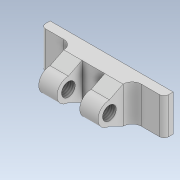
# Autodesk Inventor part: dobradicaP1
Saved by Autodesk Inventor 2020.4 (Build 244396000, 396)
## iProperties
Created: 2021-05-31
Part Number: dobradicaP1
Material: Generic
Document SubType Name: Modeling
Designer: becca
Density: 1 g/cm^3
Appearance: Default
Author: becca
Autodesk Inventor part; units mm, degrees
ref_plane "YZ Plane" through (0, 0, 0) normal (1, 0, 0) x (0, 1, 0)
ref_plane "XZ Plane" through (0, 0, 0) normal (0, 1, 0) x (-1, 0, 0)
ref_plane "XY Plane" through (0, 0, 0) normal (0, 0, 1) x (1, 0, 0)
sketch "Sketch1" plane through (0, 0, 0) normal (0, 0, 1) x (1, 0, 0)
  line L0 (0, 0) -> (27, 0)
  line L1 (27, 0) -> (27, 8)
  line L2 (27, 8) -> (0, 8)
  line L3 (0, 8) -> (0, 0)
  line L4 (5, 0) -> (22, 0)
  line L5 (22, 0) -> (22, 8)
  line L6 (22, 8) -> (5, 8)
  line L7 (5, 8) -> (5, 0)
  line L8 (7, 0) -> (20, 0)
  line L9 (20, 0) -> (20, 8)
  line L10 (20, 8) -> (7, 8)
  line L11 (7, 8) -> (7, 0)
  point P0 (7, 8)
  dimension "d0" = 27
  dimension "d1" = 8
  dimension "d2" = 17
  dimension "d3" = 13
  constraints: 24 end point, 6 parallel, 4 point on line, 3 horizontal, 3 perpendicular
  measures "d0" distance of L2.end L1.end
  measures "d1" distance of L1.end L0.end
  measures "d2" distance of L6.end L5.end
  measures "d3" distance of L10.end L9.end
extrude "Extrusion1" add sketch "Sketch1" along normal blind 2 contours L3 L2 L7 L0 | L5 L2 L1 L0
extrude "Extrusion2" add sketch "Sketch1" along normal blind 4 contours L7 L2 L11 L0 | L9 L2 L5 L0
extrude "Extrusion3" add sketch "Sketch1" along normal blind 10 contours L11 L2 L9 L0
fillet "Fillet1" radius 2 2 edges at (22, 4, 4) (5, 4, 4) inverted yes
sketch "Sketch3" plane through (20, 0, 10) normal (1, 0, 0) x (0, 0, -1)
  circle A0 centre (3, 4) radius 1.5
  circle A1 centre (3, 4) radius 2.5
  line L0 (3, 4) -> (6, 4)
  line L1 (6, 0) -> (6, 8) projected
  line L2 (3, 4) -> (3, 8)
  line L3 (6, 8) -> (0, 8) projected
  line L4 (3, 4) -> (3, 0)
  line L5 (6, 0) -> (0, 0) projected
  line L6 (3, 1.5) -> (6, 0)
  line L7 (3, 6.5) -> (6, 8)
  line L8 (0, 0) -> (0, 8) projected
  line L9 (0, 0) -> (0, 8)
  point P0 (10, 0)
  dimension "d11" = 3
  dimension "d14" = 5
  constraints: 12 end point, 3 midpoint, 2 centre point, 2 point on circle, 2 point on line, 1 coincident, 1 vertical
  measures "d11" diameter of A0
  measures "d14" diameter of A1
extrude "Extrusion4" cut sketch "Sketch3" against normal blind 20 contours L0 L2 A0 | A0 L4 L0 | L2 L4 A0 | A1 L4 L5 L8 L3 L2 | L2 L3 L7 | L6 L5 L4
sketch "Sketch5" plane through (0, 0, 0) normal (0, 0, -1) x (-1, 0, 0)
  line L0 (-20, 8) -> (-20, 0) projected
  line L1 (-20, 8) -> (-16, 8)
  line L2 (-27, 8) -> (0, 8) projected
  line L3 (-16, 8) -> (-11, 8)
  line L4 (-11, 8) -> (-7.0017, 8)
  line L5 (-16, 8) -> (-16, 0)
  line L6 (-11, 8) -> (-11, 0)
  line L7 (-16, 8) -> (-11, 8)
  line L8 (-11, 8) -> (-11, 0)
  line L9 (-11, 0) -> (-16, 0)
  line L10 (-16, 0) -> (-16, 8)
  point P0 (0, 0)
  dimension "d17" = 4
  dimension "d18" = 5
  constraints: 18 end point, 3 point on line, 2 parallel, 2 vertical, 1 horizontal, 1 perpendicular
  measures "d17" distance of L0.start L1.end
  measures "d18" distance of L1.end L3.end
extrude "Extrusion5" cut sketch "Sketch5" against normal blind 10
sketch "Sketch6" plane through (0, 0, 0) normal (0, -1, 0) x (1, 0, 0)
  line L0 (11, 0) -> (0, 0) projected
  line L1 (20, 4) -> (16, 4) projected
  line L2 (11, 0) -> (16, 0)
  line L3 (16, 0) -> (16, 4)
  line L4 (16, 4) -> (11, 4)
  line L5 (11, 4) -> (11, 0)
  constraints: 8 end point, 2 parallel, 1 horizontal, 1 perpendicular
extrude "Extrusion6" add sketch "Sketch6" against normal blind 8
fillet "Fillet2" radius 1 2 edges at (27, 4, 2) (0, 4, 2)
thread "Thread1" size "M3x0.5" class "6H" standard "ANSI Metric M Profile" full length
body "Solid1"
